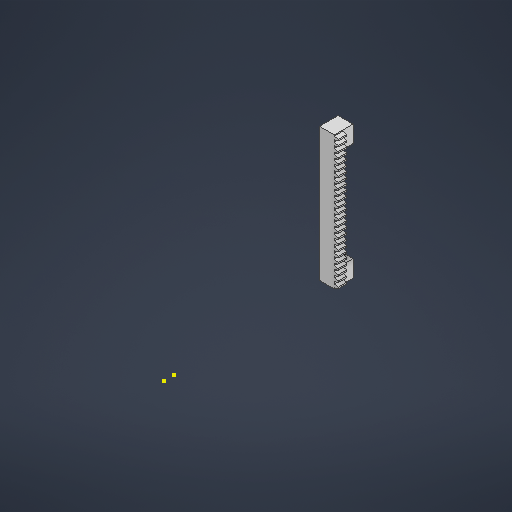
# Autodesk Inventor part: obj_2_1.齿条.STEP
Saved by Autodesk Inventor 2025 (Build 290162000, 162)
## iProperties
Created: 2026-04-25
Part Number: obj_2_1.齿条.STEP
Material: 常规
Document SubType Name: Modeling
Designer: XH
Density: 1 g/cm^3
Appearance: 默认
Author: XH
Autodesk Inventor part; units mm, degrees
ref_plane "YZ Plane" through (0, 0, 0) normal (1, 0, 0) x (0, 1, 0)
ref_plane "XZ Plane" through (0, 0, 0) normal (0, 1, 0) x (-1, 0, 0)
ref_plane "XY Plane" through (0, 0, 0) normal (0, 0, 1) x (1, 0, 0)
sketch "草图3" plane through (0, 0, 0) normal (0, 1, 0) x (-1, 0, 0)
  point P0 (0, 0)
sketch "草图4" plane through (0, 0, 0) normal (0, 0, 1) x (1, 0, 0)
  line L0 (96.7568, 180.6564) -> (96.7568, 80.6564) projected
  line L1 (99.6318, 180.6564) -> (96.7568, 180.6564) projected
  line L2 (105.5068, 180.6564) -> (102.6318, 180.6564) projected
  circle A0 centre (101.1316, 180.6563) radius 1.4998 projected
  line L3 (107.7568, 179.4984) -> (105.5068, 180.0803) projected
  line L4 (105.5068, 80.6564) -> (105.5068, 180.6564) projected
  line L5 (105.5068, 178.091) -> (107.7568, 178.6728) projected
  line L6 (107.7568, 179.4984) -> (107.7568, 178.6728) projected
  line L7 (107.7568, 176.3568) -> (107.7568, 175.5313) projected
  line L8 (107.7568, 175.5313) -> (105.5068, 174.9494) projected
  line L9 (105.5068, 176.9387) -> (107.7568, 176.3568) projected
  line L10 (105.5068, 173.7971) -> (107.7568, 173.2152) projected
  line L11 (107.7568, 173.2152) -> (107.7568, 172.3897) projected
  line L12 (107.7568, 172.3897) -> (102.5791, 171.0506) projected
  line L13 (105.5068, 170.6555) -> (107.7568, 170.0736) projected
  line L14 (107.7568, 170.0736) -> (107.7568, 169.2481) projected
  line L15 (107.7568, 169.2481) -> (105.5068, 168.6662) projected
  line L16 (105.5068, 167.5139) -> (107.7568, 166.932) projected
  line L17 (107.7568, 166.1065) -> (105.5068, 165.5246) projected
  line L18 (107.7568, 166.932) -> (107.7568, 166.1065) projected
  line L19 (105.5068, 164.3723) -> (107.7568, 163.7905) projected
  line L20 (107.7568, 163.7905) -> (107.7568, 162.9649) projected
  line L21 (107.7568, 162.9649) -> (105.5068, 162.383) projected
  line L22 (105.5068, 161.2307) -> (107.7568, 160.6488) projected
  line L23 (107.7568, 160.6488) -> (107.7568, 159.8233) projected
  line L24 (107.7568, 159.8233) -> (105.5068, 159.2414) projected
  line L25 (105.5068, 158.0892) -> (107.7568, 157.5073) projected
  line L26 (107.7568, 157.5073) -> (107.7568, 156.6817) projected
  line L27 (107.7568, 156.6817) -> (105.5068, 156.0998) projected
  line L28 (105.5068, 154.9476) -> (107.7568, 154.3657) projected
  line L29 (107.7568, 154.3657) -> (107.7568, 153.5401) projected
  line L30 (107.7568, 153.5401) -> (105.5068, 152.9582) projected
  line L31 (105.5068, 151.806) -> (107.7568, 151.2241) projected
  line L32 (107.7568, 151.2241) -> (107.7568, 150.3985) projected
  line L33 (107.7568, 150.3985) -> (105.5068, 149.8166) projected
  line L34 (105.5068, 148.6644) -> (107.7568, 148.0825) projected
  line L35 (107.7568, 148.0825) -> (107.7568, 147.2569) projected
  line L36 (107.7568, 147.2569) -> (105.5068, 146.675) projected
  line L37 (105.5068, 145.5228) -> (107.7568, 144.9409) projected
  line L38 (107.7568, 144.9409) -> (107.7568, 144.1153) projected
  line L39 (107.7568, 144.1153) -> (105.5068, 143.5334) projected
  line L40 (105.5068, 142.3812) -> (107.7568, 141.7993) projected
  line L41 (107.7568, 141.7993) -> (107.7568, 140.9737) projected
  line L42 (107.7568, 140.9737) -> (105.5068, 140.3918) projected
  line L43 (102.4905, 140.0197) -> (107.7568, 138.6577) projected
  line L44 (107.7568, 138.6577) -> (107.7568, 137.8321) projected
  line L45 (107.7568, 137.8321) -> (105.5068, 137.2503) projected
  line L46 (105.5068, 136.098) -> (107.7568, 135.5161) projected
  line L47 (107.7568, 135.5161) -> (107.7568, 134.6906) projected
  line L48 (107.7568, 134.6906) -> (105.5068, 134.1087) projected
  line L49 (105.5068, 132.9564) -> (107.7568, 132.3745) projected
  line L50 (107.7568, 132.3745) -> (107.7568, 131.549) projected
  line L51 (107.7568, 131.549) -> (105.5068, 130.9671) projected
  line L52 (105.5068, 129.8148) -> (107.7568, 129.2329) projected
  line L53 (107.7568, 129.2329) -> (107.7568, 128.4074) projected
  line L54 (107.7568, 128.4074) -> (105.5068, 127.8255) projected
  line L55 (105.5068, 126.6732) -> (107.7568, 126.0913) projected
  line L56 (107.7568, 126.0913) -> (107.7568, 125.2658) projected
  line L57 (107.7568, 125.2658) -> (105.5068, 124.6839) projected
  line L58 (105.5068, 123.5316) -> (107.7568, 122.9497) projected
  line L59 (107.7568, 122.1242) -> (102.6236, 120.7967) projected
  line L60 (107.7568, 122.9497) -> (107.7568, 122.1242) projected
  circle A1 centre (101.1329, 170.6543) radius 1.5024 projected
  circle A2 centre (101.1319, 160.6561) radius 1.5003 projected
  circle A3 centre (101.1312, 150.656) radius 1.4993 projected
  circle A4 centre (101.1297, 140.6572) radius 1.4978 projected
  circle A5 centre (101.1313, 130.6569) radius 1.4993 projected
  circle A6 centre (101.1332, 120.6547) radius 1.5023 projected
  line L61 (105.5068, 120.39) -> (107.7568, 119.8081) projected
  line L62 (107.7568, 119.8081) -> (107.7568, 118.9826) projected
  line L63 (107.7568, 118.9826) -> (105.5068, 118.4007) projected
  line L64 (105.5068, 117.2484) -> (107.7568, 116.6666) projected
  line L65 (107.7568, 116.6666) -> (107.7568, 115.841) projected
  line L66 (107.7568, 115.841) -> (105.5068, 115.2591) projected
  line L67 (105.5068, 114.1069) -> (107.7568, 113.525) projected
  line L68 (107.7568, 112.6994) -> (105.5068, 112.1175) projected
  line L69 (107.7568, 113.525) -> (107.7568, 112.6994) projected
  line L70 (105.5068, 110.9653) -> (107.7568, 110.3834) projected
  line L71 (107.7568, 110.3834) -> (107.7568, 109.5578) projected
  line L72 (107.7568, 109.5578) -> (105.5068, 108.9759) projected
  line L73 (105.5068, 104.6821) -> (107.7568, 104.1002) projected
  line L74 (107.7568, 106.4162) -> (105.5068, 105.8343) projected
  line L75 (105.5068, 107.8237) -> (107.7568, 107.2418) projected
  line L76 (107.7568, 107.2418) -> (107.7568, 106.4162) projected
  line L77 (107.7568, 104.1002) -> (107.7568, 103.2746) projected
  line L78 (107.7568, 103.2746) -> (102.0947, 101.8103) projected
  line L79 (105.5068, 101.5405) -> (107.7568, 100.9586) projected
  line L80 (107.7568, 100.9586) -> (107.7568, 100.133) projected
  line L81 (107.7568, 100.133) -> (105.5068, 99.5511) projected
  circle A7 centre (101.1318, 100.6565) radius 1.5 projected
  line L82 (105.5068, 80.6564) -> (102.6318, 80.6564) projected
  line L83 (99.6318, 80.6564) -> (96.7568, 80.6564) projected
  line L84 (96.7568, 80.6564) -> (96.7568, 180.6564) projected
  line L85 (105.5068, 92.1157) -> (107.7568, 91.5338) projected
  line L86 (107.7568, 91.5338) -> (107.7568, 90.7083) projected
  line L87 (107.7568, 90.7083) -> (105.5068, 90.1264) projected
  line L88 (107.7568, 93.8498) -> (105.5068, 93.268) projected
  line L89 (107.7568, 94.6754) -> (107.7568, 93.8498) projected
  line L90 (105.5068, 95.2573) -> (107.7568, 94.6754) projected
  line L91 (107.7568, 96.9914) -> (105.5068, 96.4095) projected
  line L92 (105.5068, 98.3989) -> (107.7568, 97.817) projected
  line L93 (107.7568, 97.817) -> (107.7568, 96.9914) projected
  line L94 (107.7568, 88.3922) -> (107.7568, 87.5667) projected
  line L95 (102.3585, 89.7883) -> (107.7568, 88.3922) projected
  circle A8 centre (101.1321, 90.6562) radius 1.5004 projected
  line L96 (107.7568, 87.5667) -> (105.5068, 86.9848) projected
  line L97 (105.5068, 85.8325) -> (107.7568, 85.2506) projected
  line L98 (107.7568, 85.2506) -> (107.7568, 84.4251) projected
  line L99 (107.7568, 84.4251) -> (105.5068, 83.8432) projected
  line L100 (105.5068, 82.6909) -> (107.7568, 82.109) projected
  line L101 (107.7568, 82.109) -> (107.7568, 81.2835) projected
  line L102 (107.7568, 81.2835) -> (105.5068, 80.7016) projected
  circle A9 centre (101.1318, 80.6565) radius 1.5 projected
  line L103 (96.7568, 80.6564) -> (105.5068, 80.6564)
  line L104 (105.5068, 80.6564) -> (105.5068, 180.6564)
  line L105 (105.5068, 180.6564) -> (96.7568, 180.6564)
  line L106 (96.7568, 180.6564) -> (96.7568, 80.6564)
  point P0 (0, 0)
  point P1 (105.5068, 171.8078)
  point P2 (102.6314, 180.6564)
  point P3 (99.6318, 180.6564)
  point P4 (99.6318, 80.6564)
  point P5 (102.6317, 80.6564)
  point P6 (105.5068, 88.9741)
  point P7 (105.5068, 102.6927)
  point P8 (105.5068, 121.5423)
  point P9 (105.5068, 139.2396)
  constraints: 8 end point, 2 parallel, 1 horizontal, 1 perpendicular, 1 other
extrude "拉伸2" add sketch "草图4" along normal blind 4 contours L1 A0 L2 L4 L82 A9 L83 L0 | L3 L6 L5 L4 | L4 L100 L101 L102 | L9 L7 L8 L4 | L4 L97 L98 L99 | L10 L11 L12 L4 | L4 L95 L94 L96 | L13 L14 L15 L4 | L4 L85 L86 L87 | L16 L18 L17 L4 | L4 L90 L89 L88 | L19 L20 L21 L4 | L4 L92 L93 L91 | L22 L23 L24 L4 | L4 L79 L80 L81 | L25 L26 L27 L4 | L4 L73 L77 L78 | L28 L29 L30 L4 | L4 L75 L76 L74 | L31 L32 L33 L4 | L4 L70 L71 L72 | L34 L35 L36 L4 | L4 L67 L69 L68 | L37 L38 L39 L4 | L4 L64 L65 L66 | L40 L41 L42 L4 | L4 L61 L62 L63 | L43 L44 L45 L4 | L4 L58 L60 L59 | L46 L47 L48 L4 | L4 L55 L56 L57 | L49 L50 L51 L4 | L4 L52 L53 L54
sketch "草图5" plane through (0, 0, 0) normal (0, 0, -1) x (-1, 0, 0)
  line L0 (-88.0523, 73.2869) -> (-124.347, 73.2869)
  line L1 (-124.347, 73.2869) -> (-124.347, 102.0841)
  line L2 (-124.347, 102.0841) -> (-88.0523, 102.0841)
  line L3 (-88.0523, 102.0841) -> (-88.0523, 73.2869)
  line L4 (-119.7058, 102.0841) -> (-61.5255, 102.0841) projected
  point P0 (0, 0)
  constraints: 8 end point, 2 parallel, 1 collinear, 1 horizontal, 1 perpendicular
extrude "拉伸3" cut sketch "草图5" against normal blind 4
sketch "草图6" plane through (0, 0, 0) normal (0, 0, -1) x (-1, 0, 0)
  line L0 (-99.6318, 180.6564) -> (-96.7568, 180.6564) projected
  line L1 (-105.5068, 173.7971) -> (-105.5068, 174.9494) projected
  line L2 (-96.7568, 180.6564) -> (-105.5068, 180.6564)
  line L3 (-105.5068, 180.6564) -> (-105.5068, 170.6564)
  line L4 (-105.5068, 170.6564) -> (-96.7568, 170.6564)
  line L5 (-96.7568, 170.6564) -> (-96.7568, 180.6564)
  line L6 (-105.5068, 180.6564) -> (-102.6314, 180.6564) projected
  line L7 (-105.5068, 102.0841) -> (-105.5068, 102.6927) projected
  line L8 (-96.7568, 180.6564) -> (-96.7568, 102.0841) projected
  line L9 (-105.5068, 102.0841) -> (-96.7568, 102.0841)
  line L10 (-96.7568, 102.0841) -> (-96.7568, 112.0841)
  line L11 (-96.7568, 112.0841) -> (-105.5068, 112.0841)
  line L12 (-105.5068, 112.0841) -> (-105.5068, 102.0841)
  line L13 (-100.6713, 102.0841) -> (-96.7568, 102.0841) projected
  point P0 (0, 0)
  point P1 (-104.0691, 180.6564)
  dimension "d6" = 10
  dimension "d7" = 10
  constraints: 16 end point, 4 parallel, 2 horizontal, 2 perpendicular, 2 point on line, 1 midpoint
  measures "d6" distance from line of point (-104.069, 180.656) L4
  measures "d7" distance between parallel lines of L13 L11
extrude "拉伸4" add sketch "草图6" along normal blind 6
delete faces "删除1" heal yes whole lump no faces at (101.4922, 102.1125, 2.6667)
delete faces "删除2" heal yes whole lump no faces at (101.0714, 179.1577, 2.6667)
delete faces "删除3" heal yes whole lump no faces at (99.6353, 170.5348, 1.3333) (102.6274, 160.5354, 2.6667) (102.0794, 151.8173, 2.6667) (102.5077, 141.2443, 2.6667) (102.5535, 130.1821, 2.6667) (101.0727, 122.1557, 2.6667)
sketch "草图7" plane through (0, 0, -6) normal (0, 0, -1) x (-1, 0, 0)
  point P0 (0, 0)
sketch "草图8" plane through (0, 0, -6) normal (0, 0, -1) x (-1, 0, 0)
  circle A0 centre (-101.3501, 175.906) radius 2
  line L0 (-105.5068, 170.6564) -> (-96.7568, 170.6564) projected
  line L1 (-105.5068, 180.6564) -> (-96.7568, 170.6564)
  line L2 (-105.5068, 112.0841) -> (-96.7568, 112.0841) projected
  line L3 (-96.7568, 102.0841) -> (-105.5068, 102.0841) projected
  line L4 (-105.5068, 112.0841) -> (-96.7568, 102.0841)
  circle A1 centre (-101.1318, 107.0841) radius 2
  point P0 (0, 0)
  dimension "d10" = 4
  dimension "d11" = 4
  constraints: 4 end point, 2 centre point, 1 coincident, 1 midpoint, 1 point on line
  measures "d10" diameter of A0
  measures "d11" diameter of A1
extrude "拉伸5" cut sketch "草图8" against normal blind 4
move faces "移动1" translate (0, 0, 1) faces at (99.6734, 138.5656, 4)
equation "\"d12\" = d10"
